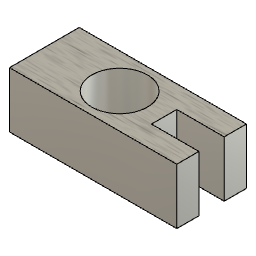
Solution 3 (Autodesk Fusion 360 design; units mm, degrees)
Autodesk Fusion 360 part; units mm, degrees
sketch "Sketch1" plane through (0, 0, 0) normal (0, 1, 0) x (1, 0, 0)
  line L0 (0, 0) -> (0, -25)
  line L1 (0, 0) -> (60, 0)
  line L2 (0, -25) -> (60, -25)
  line L3 (60, -17.0662) -> (43, -17.0662)
  circle A0 centre (27, -12.5) radius 10
  line L4 (60, -25) -> (60, -17)
  line L5 (60, 0) -> (60, -8)
  line L6 (60, -8) -> (43, -8)
  line L7 (43, -8) -> (43, -17.0662)
  dimension "d1" = 25
  dimension "d2" = 60
  dimension "d3" = 60
  dimension "d21" = 20
  constraint coincident L0.start L1.start
  constraint vertical L0
  constraint perpendicular L0 L1
  constraint perpendicular L0 L2
  constraint perpendicular L3 L4
  constraint perpendicular L1 L5
  constraint perpendicular L5 L6
  constraint perpendicular L3 L7
  measures "d1" distance of L0.start L0.end
  measures "d2" distance of L0.start L1.end
  measures "d3" distance of L0.end L2.end
  measures "d21" diameter of A0
extrude "Extrude1" add sketch "Sketch1" along normal blind 5 contours L0 L1 L2 L3 L4 L5 L6 L7 | A0
extrude "Extrude2" cut 1 faces at (14.3333, 5, 11) along direction (0, -1, 0) blind 5
extrude "Extrude3" add sketch "Sketch1" along normal blind 20
